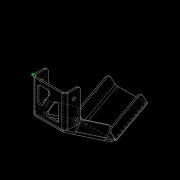
# Autodesk Inventor part: HipCoverTop
Saved by Autodesk Inventor 2020 (Build 240168000, 168)
## iProperties
Created: 2020-05-25
Part Number: HipCoverTop
Material: Generic
Document SubType Name: Sheet Metal
Designer: valer
Density: 1 g/cm^3
Sheet Metal Rule: Default
Appearance: Default
Author: valer
Autodesk Inventor part; units mm, degrees
ref_plane "YZ Plane" through (0, 0, 0) normal (1, 0, 0) x (0, 1, 0)
ref_plane "XZ Plane" through (0, 0, 0) normal (0, 1, 0) x (-1, 0, 0)
ref_plane "XY Plane" through (0, 0, 0) normal (0, 0, 1) x (1, 0, 0)
sketch "Base" plane through (0, 0, 0) normal (0, 0, 1) x (1, 0, 0)
  line L0 (0, 0) -> (34.29, 0)
  line L1 (34.29, 0) -> (34.29, -65.2018)
  line L2 (34.29, -65.2018) -> (0, -65.2018)
  line L3 (0, -65.2018) -> (0, 0)
  dimension "d0" = 65.2018
  dimension "d1" = 34.29
  measures "d0" distance of L2.end L0.start
  measures "d1" distance of L0.start L0.end
extrude "Plate1" add sketch "Base" along normal blind 3.048
sketch "Sketch2" plane through (3.048, 0, 3.048) normal (-1, 0, 0) x (0, -1, 0)
  line L0 (65.2018, 0) -> (0, 0)
  line L1 (0, 0) -> (0, -31.75)
  line L2 (0, -31.75) -> (65.2018, -31.75)
  line L3 (65.2018, -31.75) -> (65.2018, 0)
  constraints: 6 end point, 1 horizontal, 1 perpendicular, 1 vertical
edge flange "MountFeature" height 31.75 angle 90 thickness 3.048 bend radius 3.048 thickness toward (-1, 0, 0) relief straight relief width 3.048 relief depth 1.524 edges at (0, -32.6009, 0) wall of the first edge with corners at (3.048, -65.2018, 3.048) (3.048, 0, 3.048) (3.048, 0, -28.702) (3.048, -65.2018, -28.702)
bend "Bend1"
corner "Corner1"
sketch "MountHoles" plane through (0, -65.2018, -28.702) normal (-1, 0, 0) x (0, 0, 1)
  arc A0 (10.150845, 50.036867) -> (15.493805, 46.605354) centre (12.822325, 48.32111) ccw
  arc A1 (7.802732, 11.528906) -> (5.106142, 5.779914) centre (6.454437, 8.65441) ccw
hole "MountHolesFeature" at (0, -16.88069, -15.879675) at (0, -56.54739, -22.247563) direction (1, 0, 0) diameter 6.35 end through all
mirror "Mirror1" about plane through (34.29, 0, 0) normal (1, 0, 0)
sketch "Sketch4" plane through (0, 0, 3.048) normal (0, 0, 1) x (1, 0, 0)
  line L0 (12.7, -8.466667) -> (12.7, -56.735133)
  line L1 (12.7, -56.735133) -> (41.139516, -8.466667)
  line L2 (41.139516, -8.466667) -> (12.7, -8.466667)
  line L3 (62.484, 0) -> (6.096, 0)
  line L4 (27.440484, -56.735133) -> (55.88, -8.466667)
  line L5 (55.88, -8.466667) -> (55.88, -56.735133)
  line L6 (55.88, -56.735133) -> (27.440484, -56.735133)
  line L7 (41.139516, -8.466667) -> (55.88, -8.466667) construction
  line L8 (12.7, -56.735133) -> (27.440484, -56.735133) construction
  line L9 (0, -65.2018) -> (0, 0)
  line L10 (68.58, -65.2018) -> (68.58, 0)
  line L11 (62.484, -65.2018) -> (6.096, -65.2018)
  dimension "d23" = 8.46667
  dimension "d24" = 12.7
  dimension "d25" = 12.7
  dimension "d26" = 8.46667
  dimension "d27" = 12.7
  constraints: 16 end point, 2 parallel, 2 perpendicular, 1 collinear, 1 horizontal, 1 vertical
  measures "d23" distance between parallel lines of L3 L2
  measures "d24" distance between parallel lines of L9 L0
  measures "d25" distance between parallel lines of L5 L10
  measures "d26" distance between parallel lines of L11 L6
  measures "d27" distance between parallel lines of L4 L1
extrude "Extrusion1" cut sketch "Sketch4" against normal blind 25.4
fillet "Fillet2" radius 5.08 6 edges at (12.7, -8.4667, 1.524) (12.7, -56.7351, 1.524) (41.1395, -8.4667, 1.524) (55.88, -8.4667, 1.524) (27.4405, -56.7351, 1.524) (55.88, -56.7351, 1.524)
sketch "Sketch5" plane through (62.484, -67.724236, -1.33697) normal (0, -0.8275708, 0.5613614) x (1, 0, 0)
  line L0 (-56.388, 0) -> (0, 0)
  line L1 (0, 0) -> (0, 118.688928)
  line L2 (0, 118.688928) -> (-56.388, 118.688928)
  line L3 (-56.388, 118.688928) -> (-56.388, 0)
  constraints: 6 end point, 1 horizontal, 1 perpendicular, 1 vertical
edge flange "Flange2" height 121.92 angle 55.85 thickness 3.048 bend radius 3.048 thickness toward (0, -0.8275708, 0.5613614) relief straight relief width 3.048 relief depth 1.524 edges at (34.29, -65.2018, 3.048) wall of the first edge with corners at (6.096, -67.724236, -1.33697) (62.484, -67.724236, -1.33697) (62.484, -134.351618, -99.560458) (6.096, -134.351618, -99.560458)
bend "Bend2"
corner "Corner2"
sketch "Sketch6" plane through (6.096, -134.519407, -102.704315) normal (0, -0.8826196, -0.4700879) x (1, 0, 0)
  line L0 (56.388, 0) -> (0, 0)
  line L1 (0, 0) -> (0, -72.523383)
  line L2 (0, -72.523383) -> (56.388, -72.523383)
  line L3 (56.388, -72.523383) -> (56.388, 0)
  constraints: 6 end point, 1 horizontal, 1 perpendicular, 1 vertical
edge flange "Flange3" height 76.2 angle 62.19 thickness 3.048 bend radius 3.048 thickness toward (0, -0.8826196, -0.4700879) relief straight relief width 3.048 relief depth 1.524 edges at (34.29, -134.351618, -99.560458) wall of the first edge with corners at (62.484, -134.519407, -102.704315) (6.096, -134.519407, -102.704315) (6.096, -100.427045, -166.714876) (62.484, -100.427045, -166.714876)
bend "Bend3"
corner "Corner3"
sketch "Sketch8" plane through (3.048, -131.829183, -101.271487) normal (-1, 0, 0) x (0, -1, 0)
  line L0 (-34.092362, -64.010561) -> (0, 0)
  line L1 (0, 0) -> (-22.642724, 12.059634)
  line L2 (-22.642724, 12.059634) -> (-56.735086, -51.950927)
  line L3 (-56.735086, -51.950927) -> (-34.092362, -64.010561)
  constraints: 6 end point, 1 perpendicular, 2 other
edge flange "Flange4" height 31.75 angle 90 thickness 3.048 bend radius 3.048 thickness toward (-1, 0, 0) relief straight relief width 3.048 relief depth 1.524 corner gap 3.048 corner form 0 edges at (6.096, -117.473226, -134.709596) (62.484, -117.473226, -134.709596) wall of the first edge with corners at (3.048, -97.736821, -165.282049) (3.048, -131.829183, -101.271487) (3.048, -109.186459, -89.211853) (3.048, -75.094097, -153.222415)
bend "Bend4"
corner "Corner4"
fillet "OutsideFilletsFeature" radius 6.35 8 edges at (1.524, -65.2018, -28.702) (1.524, 0, -28.702) (1.524, -109.1865, -89.2119) (67.056, -75.0941, -153.2224) (1.524, -75.0941, -153.2224) (67.056, -109.1865, -89.2119) (67.056, -65.2018, -28.702) (67.056, 0, -28.702)
sketch "Sketch10" plane through (6.096, -70.246671, 0.374059) normal (0, -0.8275708, 0.5613614) x (1, 0, 0)
  line L0 (-3.048, -18.760781) -> (-6.096, -18.760781)
  line L1 (-3.048, -98.227084) -> (-6.096, -98.227084)
  line L2 (-6.096, -21.300781) -> (0, -21.300781)
  line L3 (0, -21.300781) -> (0, -95.687084)
  line L4 (0, -95.687084) -> (-6.096, -95.687084)
  line L5 (-6.096, -95.687084) -> (-6.096, -21.300781)
  line L6 (-6.096, 0) -> (-6.096, -15.975426)
  line L7 (0, 0) -> (0, -118.688928)
  point P0 (-6.096, 39.124209)
  dimension "d65" = 2.54
  dimension "d66" = 2.54
  measures "d65" distance between parallel lines of L0 L2
  measures "d66" distance between parallel lines of L1 L4
sheet face with bend "Face2" sketch "Sketch10" thickness 3.048 toward (0, 0.8275708, -0.5613614) bend radius 3.048 relief straight relief width 3.048 relief depth 1.524
bend "Bend5"
sketch "Sketch11" plane through (3.048, -82.204108, -17.253845) normal (-1, 0, 0) x (0, -1, 0)
  line L0 (41.757599, -61.55993) -> (0, 0)
  line L1 (0, 0) -> (-21.020298, -14.25858)
  line L2 (-21.020298, -14.25858) -> (20.737301, -75.818509)
  line L3 (20.737301, -75.818509) -> (41.757599, -61.55993)
  constraints: 6 end point, 1 perpendicular, 2 other
edge flange "Flange5" height 25.4 angle 90 thickness 3.048 bend radius 3.048 thickness toward (-1, 0, 0) relief straight relief width 3.048 relief depth 1.524 edges at (0, -100.560472, -49.744839) wall of the first edge with corners at (3.048, -123.961707, -78.813774) (3.048, -82.204108, -17.253845) (3.048, -61.18381, -31.512424) (3.048, -102.941409, -93.072354)
bend "Bend6"
corner "Corner5"
ref_plane "MiddlePlane" through (34.29, -97.736821, -165.282049) normal (-1, 0, 0) x (0, -0.4700879, 0.8826196)
mirror "Mirror2" about plane through (34.29, -97.736821, -165.282049) normal (-1, 0, 0) of "Flange5"
fillet "Fillet3" radius 6.35 4 edges at (1.524, -102.9414, -93.0724) (67.056, -102.9414, -93.0724) (1.524, -61.1838, -31.5124) (67.056, -61.1838, -31.5124)
sketch "Sketch12" plane through (0, -97.736821, -165.282049) normal (-1, 0, 0) x (0, -0.4700879, 0.8826196)
  arc A0 (30.823709, 17.304472) -> (24.557799, 18.334458) centre (27.690754, 17.819465) ccw
  arc A1 (68.203567, 17.535556) -> (62.188704, 15.499893) centre (65.196135, 16.517724) ccw
  point P0 (99.936287, 163.961521)
hole "Hole2" at (0, -113.805865, -99.973878) at (0, -95.026098, -132.464931) direction (1, 0, 0) diameter 6.35 end through all
equation "\"d20\" = Thickness"
equation "\"d25\" = d24"
equation "\"d26\" = d23"
equation "\"d27\" = d24"
equation "\"d66\" = d65"
equation "\"d88\" = Thickness"
equation "\"d2\" = Thickness"
equation "\"d3\" = BendReliefWidth"
equation "\"d4\" = BendReliefDepth"
equation "\"d5\" = MinimumRemnant"
equation "\"d6\" = TransitionRadius"
equation "\"d9\" = BendRadius"
equation "\"d10\" = CornerReliefSize"
equation "\"d11\" = GapSize"
equation "\"d12\" = JacobiRadiusSize"
equation "\"d31\" = BendReliefWidth"
equation "\"d32\" = BendReliefDepth"
equation "\"d33\" = MinimumRemnant"
equation "\"d34\" = TransitionRadius"
equation "\"d37\" = BendRadius"
equation "\"d38\" = CornerReliefSize"
equation "\"d39\" = GapSize"
equation "\"d40\" = JacobiRadiusSize"
equation "\"d41\" = BendReliefWidth"
equation "\"d42\" = BendReliefDepth"
equation "\"d43\" = MinimumRemnant"
equation "\"d44\" = TransitionRadius"
equation "\"d47\" = BendRadius"
equation "\"d48\" = CornerReliefSize"
equation "\"d49\" = GapSize"
equation "\"d50\" = JacobiRadiusSize"
equation "\"d51\" = BendReliefWidth"
equation "\"d52\" = BendReliefDepth"
equation "\"d53\" = MinimumRemnant"
equation "\"d54\" = TransitionRadius"
equation "\"d57\" = BendRadius"
equation "\"d58\" = CornerReliefSize"
equation "\"d59\" = GapSize"
equation "\"d60\" = JacobiRadiusSize"
equation "\"d67\" = BendRadius"
equation "\"d68\" = BendReliefWidth"
equation "\"d70\" = MinimumRemnant"
equation "\"d69\" = BendReliefDepth"
equation "\"d71\" = TransitionRadius"
equation "\"d72\" = BendReliefWidth"
equation "\"d73\" = BendReliefDepth"
equation "\"d74\" = MinimumRemnant"
equation "\"d75\" = TransitionRadius"
equation "\"d78\" = BendRadius"
equation "\"d79\" = CornerReliefSize"
equation "\"d80\" = GapSize"
equation "\"d81\" = JacobiRadiusSize"
equation "\"BendRadius\" = Thickness"
equation "\"BendReliefWidth\" = Thickness"
equation "\"BendReliefDepth\" = 0.5 * Thickness"
equation "\"CornerReliefSize\" = 4 * Thickness"
equation "\"MinimumRemnant\" = 2 * Thickness"
equation "\"TransitionRadius\" = BendRadius"
equation "\"JacobiRadiusSize\" = BendRadius"
equation "\"GapSize\" = Thickness"
equation "\"Thickness\" = 3.048"
body "Solid1"
